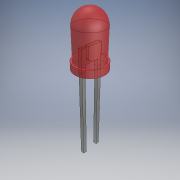
# Autodesk Inventor part: LED-5mm-Red
Saved by Autodesk Inventor 2018 (Build 220112000, 112)
## iProperties
Created: 2021-02-02
Part Number: LED-5mm-Red
Material: Všeobecné
Document SubType Name: Modeling
Designer: Jozko Mrkvicka
Density: 1 g/cm^3
Appearance: Výchozí
Author: Jozko Mrkvicka
Autodesk Inventor part; units mm, degrees
sketch "Náčrt1" plane through (0, 0, 0) normal (0, 1, 0) x (-1, 0, 0)
  circle A0 centre (0, 0) radius 2.8575
  dimension "d0" = 5.715
  constraints: 1 centre point
  measures "d0" diameter of A0
extrude "Vysunutí1" add sketch "Náčrt1" along normal blind 1.27
sketch "Náčrt2" plane through (0, 1.27, 0) normal (0, 1, 0) x (1, 0, 0)
  circle A0 centre (0, 0) radius 2.8575 projected
  circle A1 centre (0, 0) radius 2.54
  dimension "d3" = 5.08
  constraints: 1 centre point, 1 coincident
  measures "d3" diameter of A1
extrude "Vysunutí2" add sketch "Náčrt2" along normal blind 7.62 contours A1
fillet "Zaoblení1" radius 2.54 1 edges at (-2.54, 8.89, 0)
ref_plane "Pracovní rovina1" through (0, 0, 0) normal (0, -1, 0) x (1, 0, 0)
ref_plane "Pracovní rovina3" through (0, 0.635, 0) normal (0, -1, 0) x (1, 0, 0)
sketch "Náčrt6" plane through (0, 0.635, 0) normal (0, -1, 0) x (1, 0, 0)
  line L0 (20.2707, 4.967) -> (20.2707, -12.8191)
  line L1 (20.2707, -12.8191) -> (20.9057, -12.8191)
  line L2 (17.7307, -12.8191) -> (17.0957, -12.8191)
  line L3 (17.0957, -12.8191) -> (17.0957, 7.4969)
  line L4 (20.2707, 4.967) -> (19.0001, 4.967)
  line L5 (19.0001, 4.967) -> (18.3771, 5.5899)
  line L6 (20.9057, 7.4969) -> (18.3771, 7.4969)
  line L7 (18.3771, 7.4969) -> (18.3771, 5.5899)
  line L8 (17.7307, 4.967) -> (18.6299, 4.967)
  line L9 (18.6299, 4.967) -> (17.9883, 5.6086)
  line L10 (17.0957, 7.4969) -> (17.9883, 7.4969)
  line L11 (17.9883, 7.4969) -> (17.9883, 5.6086)
  line L12 (20.9057, -12.8191) -> (20.9057, 7.4969)
  line L13 (17.7307, 4.967) -> (17.7307, -12.8191)
  point P0 (0, 0)
  dimension "d36" = 135
  constraints: 28 end point, 4 horizontal, 3 perpendicular, 2 vertical
  measures "d36" angle of L4 L5
extrude "Vysunutí5" add sketch "Náčrt6" along normal blind 0.635
ref_plane "Pracovní rovina4" through (17.0957, 0.3175, -12.8191) normal (-1, 0, 0) x (0, 0, 1)
split body "Rozdělit2" result two bodies by plane through (17.0957, 0.3175, -12.8191) normal (-1, 0, 0) first body at (2.0334, 4.6567, 0.1642)
move or copy body "Posunout těleso9" bodies to move or copy 3 copy no rotation origin (0, 0, 0) rotation axis (1, 0, 0) rotation angle -90 translate (0, -6.8619, 8.1319)
move or copy body "Posunout těleso10" bodies to move or copy 3 copy no translate (-18.9992, 3.048, -7.7978)
combine bodies "Kombinovat1" operation type subtract main body 2 bodies to subtract 3 keep tools yes
